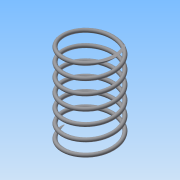
# Autodesk Inventor part: пружина т8
Saved by Autodesk Inventor 2017 (Build 210142000, 142)
## iProperties
Part Number: пружина т8
Material: Типовые
Document SubType Name: Modeling
Designer: Max
Mass: 0.111979 g
Surface Area: 5.72893 cm^2
Volume: 0.111979 cm^3
Density: 1 g/cm^3
Appearance: Сталь — полированная
Author: Max
Autodesk Inventor part; units mm, degrees
ref_plane "YZ Plane" through (0, 0, 0) normal (1, 0, 0) x (0, 1, 0)
ref_plane "XZ Plane" through (0, 0, 0) normal (0, 1, 0) x (-1, 0, 0)
ref_plane "XY Plane" through (0, 0, 0) normal (0, 0, 1) x (1, 0, 0)
sketch "Эскиз1" plane through (0, 0, 0) normal (1, 0, 0) x (0, 1, 0)
  line L0 (0, 0) -> (0, 122.0283) construction
  circle A0 centre (5.6, 0) radius 0.4
  line L1 (0, 0) -> (0, 20)
  line L2 (0, 20) -> (15.1384, 20)
  dimension "d0" = 0.8
  dimension "d1" = 6
  dimension "d2" = 5.2
  dimension "d11" = 20
  constraints: 6 end point, 1 centre point, 1 perpendicular, 1 point on line, 1 vertical
  measures "d0" diameter of A0
  measures "d2" distance edge to line of A0 L0
  measures "d11" distance of L0.start L1.end
coil "Пружина1" sketch "Эскиз1" operation add axis through (0, 0, 0) along (0, 0, 1) pitch 3 turns 12 hand right
sketch "Эскиз2" plane through (0, 0, 0) normal (1, 0, 0) x (0, 1, 0)
  line L0 (15.4563, 7.1627) -> (-18.1706, 7.1627)
  line L1 (-18.1706, 7.1627) -> (-18.1706, -9.9524)
  line L2 (-18.1706, -9.9524) -> (15.4563, -9.9524)
  line L3 (15.4563, -9.9524) -> (15.4563, 7.1627)
  line L4 (14.7778, 49.6111) -> (-18.1706, 49.6111)
  line L5 (-18.1706, 49.6111) -> (-18.1706, 26.1627)
  line L6 (-18.1706, 26.1627) -> (14.7778, 26.1627)
  line L7 (14.7778, 26.1627) -> (14.7778, 49.6111)
  point P0 (0, 0)
  dimension "d12" = 19
  constraints: 16 end point, 4 parallel, 2 horizontal, 2 perpendicular
  measures "d12" distance between parallel lines of L0 L6
extrude "Выдавливание1" cut sketch "Эскиз2" along normal mid plane 30
